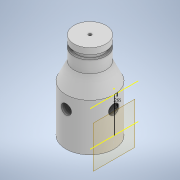
# Autodesk Inventor part: piston badflowchannel-1-16in-thread
Saved by Autodesk Inventor 2020 (Build 240168000, 168)
## iProperties
Created: 2022-01-16
Part Number: piston badflowchannel-1-16in-thread
Material: Generic
Document SubType Name: Modeling
Designer: pab2
Density: 1 g/cm^3
Appearance: Default
Author: pab2
Autodesk Inventor part; units mm, degrees
ref_plane "YZ Plane" through (0, 0, 0) normal (1, 0, 0) x (0, 1, 0)
ref_plane "XZ Plane" through (0, 0, 0) normal (0, 1, 0) x (-1, 0, 0)
ref_plane "XY Plane" through (0, 0, 0) normal (0, 0, 1) x (1, 0, 0)
sketch "Sketch1" plane through (0, 0, 0) normal (0, 0, 1) x (1, 0, 0)
  line L0 (0, 0) -> (8.4519, 0)
  line L1 (8.4519, 0) -> (8.4519, 12.7)
  line L2 (8.4519, 12.7) -> (7.0041, 12.7)
  line L3 (7.0041, 12.7) -> (7.0041, 15.113)
  line L4 (7.0041, 15.113) -> (8.4519, 15.113)
  line L5 (8.4519, 15.113) -> (8.4519, 18.288)
  line L6 (8.4519, 18.288) -> (0, 18.288)
  line L7 (0, 18.288) -> (0, 0)
  line L8 (0, -29.2334) -> (0, 26.2082) projected
  line L9 (8.4519, 0) -> (8.4519, 6.35)
  line L10 (8.4519, 0) -> (8.4519, 6.35)
  line L11 (8.4519, 6.35) -> (15.4293, -8.6131)
  line L12 (8.4519, 6.35) -> (24.9619, 6.35) construction
  line L13 (15.4293, -8.6131) -> (12.2543, -8.6131)
  line L14 (12.2543, -8.6131) -> (8.4519, 0)
  line L15 (15.4293, -8.6131) -> (0, -8.6131)
  line L16 (0, 0) -> (8.4519, 0)
  line L17 (0, -8.6131) -> (12.7, -8.6131)
  line L18 (12.7, -8.6131) -> (12.7, -21.3131)
  line L19 (12.7, -21.3131) -> (0, -21.3131)
  line L20 (0, -21.3131) -> (0, -8.6131)
  line L21 (12.7, -8.6131) -> (12.7, -2.7602)
  point P0 (12.2543, -8.6131)
  dimension "d0" = 8.4519
  dimension "d1" = 12.7
  dimension "d2" = 90
  dimension "d3" = 1.4478
  dimension "d4" = 2.413
  dimension "d5" = 3.175
  dimension "d23" = 16.51
  dimension "d24" = 65
  dimension "d25" = 3.175
  dimension "d83" = 12.7
  dimension "d84" = 12.7
  constraints: 42 end point, 8 perpendicular, 4 point on line, 3 horizontal, 3 parallel, 2 vertical, 1 collinear, 1 equal length, 1 midpoint
  measures "d0" distance of L0.start L0.end
  measures "d1" distance of L0.end L1.end
  measures "d2" angle of L1 L0
  measures "d3" distance of L1.end L2.end
  measures "d4" distance of L2.end L3.end
  measures "d5" distance of L4.end L5.end
  measures "d23" distance of L9.end L11.end
  measures "d24" angle of L11 L12
  measures "d25" distance of L11.end L13.end
  measures "d83" distance of L18.end L19.end
  measures "d84" distance of L17.end L18.end
revolve "Revolution1" add sketch "Sketch1" angle 360 about axis through (0, -10, 0) along (0, 1, 0) contours L7 L6 L5 L4 L3 L2 L1 L0 | L0 L14 L15 L8 | L1 L11 L21 L13 L14 | L15 L13 L18 L19 L8
sketch "Sketch12" plane through (0, 18.288, 0) normal (0, 1, 0) x (1, 0, 0)
  point P0 (0, 0)
  point P1 (0, 0)
  constraints: 1 coincident
hole "Hole4" at (0, 18.288, 0) direction (0, -1, 0) diameter 1.5875 depth 32.8676 tip angle 118
sketch "Sketch13" plane through (0, -21.3131, 0) normal (0, -1, 0) x (1, 0, 0)
  circle A0 centre (0, 0) radius 12.7 projected
  point P0 (12.7, 0)
  point P1 (0, -12.7)
  point P2 (-12.7, 0)
  point P3 (0, 12.7)
  constraints: 4 point on circle
ref_plane "Work Plane1" through (12.7, -21.3131, 0) normal (1, 0, 0) x (0, 1, 0)
sketch "Sketch14" plane through (12.7, -21.3131, 0) normal (1, 0, 0) x (0, 1, 0)
  line L0 (0, 12.7) -> (0, -12.7) projected
  line L1 (0, 0) -> (18.553, 0)
  line L2 (18.553, 12.7) -> (18.553, -12.7) projected
  line L3 (18.553, 0) -> (11.8347, 0)
  point P0 (21.3131, 0)
  dimension "d92" = 6.7183
  constraints: 4 end point, 2 midpoint, 1 point on line
  measures "d92" distance of L1.end L3.end
hole "Hole5" at (12.7, -9.4785, 0) direction (-1, 0, 0) diameter 1.5875 end through all
hole "Hole6" at (12.7, -9.4785, 0) direction (-1, 0, 0) diameter 5.3594 depth 6.35 thread size "1/4-28 UNF" class "2B" standard "ANSI Unified Screw Threads"
extrude "Extrusion3" add sketch "Sketch13" along normal blind 6.35
sketch "Sketch16" plane through (0, -27.6631, 0) normal (0, -1, 0) x (1, 0, 0)
  point P0 (0, 0)
hole "Hole8" at (0, -27.6631, 0) direction (0, 1, 0) diameter 4.9784 depth 6.35 thread size "1/4-20 UNC" class "2B" standard "ANSI Unified Screw Threads"
pattern_circular "Circular Pattern5" count 4 over 360 about axis through (0, -10, 0) along (0, 1, 0) of "Hole5", "Hole6"
equation "\"d54\" = 55deg"
equation "\"Sketch7_Pitch\" = 0.90714"
equation "\"d72\" = 55deg"
equation "\"Sketch9_Pitch\" = 1.27"
equation "\"d137\" = 55deg"
equation "\"Sketch17_Pitch\" = 1.27"
equation "\"d155\" = 55deg"
equation "\"Sketch19_Pitch\" = 0.90714"
equation "\"d173\" = 55deg"
equation "\"Sketch21_Pitch\" = 0.90714"
equation "\"d191\" = 55deg"
equation "\"Sketch23_Pitch\" = 1.27"
equation "\"d221\" = 55deg"
equation "\"Sketch25_Pitch\" = 0.90714"
equation "\"d239\" = 55deg"
equation "\"Sketch27_Pitch\" = 1.27"
body "Solid1"
